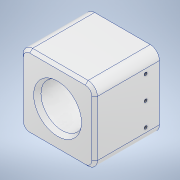
# Autodesk Inventor part: Temperierblock
Saved by Autodesk Inventor 2021 (Build 250183000, 183)
## iProperties
Created: 2021-04-25
Part Number: Temperierblock
Material: Aluminium 6061
Document SubType Name: Modeling
Designer: Sebastian Seewald
Density: 2.7 g/cm^3
Appearance: Aluminium - flach
Mass: 877.287 g
Surface Area: 506.723 cm^2
Volume: 324.921 cm^3
Author: Sebastian Seewald
Autodesk Inventor part; units mm, degrees
note: some values were not read from the file. Chosen so that the rebuilt part matches the saved one: pattern direction of "Rechteckige Anordnung1".
ref_plane "YZ Plane" through (0, 0, 0) normal (1, 0, 0) x (0, 1, 0)
ref_plane "XZ Plane" through (0, 0, 0) normal (0, 1, 0) x (-1, 0, 0)
ref_plane "XY Plane" through (0, 0, 0) normal (0, 0, 1) x (1, 0, 0)
sketch "Skizze1" plane through (0, 0, 0) normal (0, 0, 1) x (1, 0, 0)
  line L0 (-40, 40) -> (40, 40)
  line L1 (40, 40) -> (40, -40)
  line L2 (40, -40) -> (-40, -40)
  line L3 (-40, -40) -> (-40, 40)
  line L4 (-40, 40) -> (40, -40) construction
  line L5 (40, 40) -> (-40, -40) construction
  point P0 (0, 0)
  dimension "d0" = 80
  dimension "d1" = 80
  constraints: 12 end point, 2 midpoint, 2 parallel, 1 horizontal, 1 perpendicular
  measures "d0" distance of L0.start L0.end
  measures "d1" distance of L2.end L0.start
extrude "Extrusion1" add sketch "Skizze1" along normal blind 70
sketch "Skizze2" plane through (0, 0, 70) normal (0, 0, 1) x (1, 0, 0)
  circle A0 centre (0, 0) radius 22.95
  dimension "d4" = 45.9
  constraints: 1 centre point, 1 coincident
  measures "d4" diameter of A0
extrude "Extrusion2" cut sketch "Skizze2" against normal blind 60
chamfer "Fase1" distance 5 angle 30 1 edges at (-22.95, 0, 70) measured on face at (22.8756, -1.8467, 30)
fillet "Rundung2" radius 10 4 edges at (40, -40, 35) (40, 40, 35) (-40, -40, 35) (-40, 40, 35)
sketch "Skizze4" plane through (0, 0, 0) normal (0, 0, -1) x (-1, 0, 0)
  line L0 (40, 30) -> (40, -30) projected
  line L1 (-30, 40) -> (30, 40) projected
  point P0 (0, 0)
  point P1 (33, 33)
  dimension "d38" = 7
  dimension "d39" = 7
  measures "d38" distance from line of point (33, 33) L0
  measures "d39" distance from line of L1 point (33, 33)
hole "Bohrung1" at (-33, 33, 0) direction (0, 0, 1) diameter 3.242 depth 18 tip angle 118 thread size "M4x0.7" class "6H" standard "ISO Metric profile"
pattern_linear "Rechteckige Anordnung1" count 2 spacing 66 along (1, 0, 0) count 2 spacing 66 along (0, -1, 0) of "Bohrung1" first direction both ways yes
chamfer "Fase2" distance 3 angle 45 8 edges at (0, -40, 70) (37.0711, -37.0711, 70) (40, 0, 70) (37.0711, 37.0711, 70) (0, 40, 70) (-37.0711, 37.0711, 70) (-40, 0, 70) (-37.0711, -37.0711, 70)
sketch "Skizze8" plane through (0, 0, 0) normal (0, 0, -1) x (-1, 0, 0)
  point P0 (0, 0)
  point P1 (-25, -25)
  point P2 (-25, 25)
  point P3 (25, 25)
  point P4 (25, -25)
  dimension "d75" = 25
  dimension "d76" = 25
  dimension "d84" = 25
  dimension "d85" = 25
  dimension "d86" = 25
  dimension "d87" = 25
  dimension "d88" = 25
  dimension "d89" = 25
  measures "d75" horizontal distance of point (0, 0) point (-25, -25)
  measures "d76" horizontal distance of point (0, 0) point (-25, -25)
  measures "d84" horizontal distance of point (0, 0) point (-25, 25)
  measures "d85" horizontal distance of point (0, 0) point (-25, 25)
  measures "d86" horizontal distance of point (0, 0) point (25, 25)
  measures "d87" horizontal distance of point (0, 0) point (25, 25)
  measures "d88" horizontal distance of point (0, 0) point (25, -25)
  measures "d89" horizontal distance of point (0, 0) point (25, -25)
hole "Bohrung3" at (25, -25, 0) at (25, 25, 0) at (-25, 25, 0) at (-25, -25, 0) direction (0, 0, 1) diameter 8 depth 60 tip angle 118
sketch "Skizze10" plane through (0, 0, 0) normal (0, 0, -1) x (-1, 0, 0)
  point P0 (0, 0)
  point P1 (-30, 0)
  point P2 (30, 0)
  dimension "d97" = 30
  dimension "d98" = 30
  constraints: 2 horizontal alignment
  measures "d97" distance of point (0, 0) point (-30, 0)
  measures "d98" distance of point (0, 0) point (30, 0)
hole "Bohrung5" at (30, 0, 0) at (-30, 0, 0) direction (0, 0, 1) diameter 5.1 depth 50 tip angle 118
sketch "Skizze12" plane through (40, -30, 0) normal (1, 0, 0) x (0, 0, -1)
  point P0 (0, 30)
  point P1 (-15, 5)
  point P2 (-15, 55)
  dimension "d108" = 25
  dimension "d109" = 25
  dimension "d110" = 15
  dimension "d111" = 15
  measures "d108" vertical distance of point (0, 30) point (-15, 5)
  measures "d109" vertical distance of point (0, 30) point (-15, 55)
  measures "d110" horizontal distance of point (0, 30) point (-15, 5)
  measures "d111" horizontal distance of point (0, 30) point (-15, 55)
hole "Bohrung6" at (40, -25, 15) at (40, 25, 15) direction (-1, 0, 0) diameter 3.242 depth 13 tip angle 118 thread size "M4x0.7" class "6H" standard "ISO Metric profile"
sketch "Skizze13" plane through (-40, -30, 0) normal (-1, 0, 0) x (0, 0, 1)
  point P0 (0, 30)
  point P1 (15, 55)
  point P2 (15, 5)
  dimension "d119" = 25
  dimension "d120" = 25
  dimension "d121" = 15
  dimension "d122" = 15
  measures "d119" vertical distance of point (0, 30) point (15, 55)
  measures "d120" vertical distance of point (0, 30) point (15, 5)
  measures "d121" horizontal distance of point (0, 30) point (15, 5)
  measures "d122" horizontal distance of point (0, 30) point (15, 55)
hole "Bohrung7" at (-40, 25, 15) at (-40, -25, 15) direction (1, 0, 0) diameter 3.242 depth 13 tip angle 118 thread size "M4x0.7" class "6H" standard "ISO Metric profile"
sketch "Skizze14" plane through (-40, -30, 0) normal (-1, 0, 0) x (0, 0, 1)
  point P0 (0, 30)
  point P1 (15, 30)
  dimension "d130" = 15
  dimension "d131" = 0
  measures "d130" distance of point (0, 30) point (15, 30)
  measures "d131" vertical distance of point (0, 30) point (15, 30)
hole "Bohrung8" at (-40, 0, 15) direction (1, 0, 0) diameter 3.242 depth 10 tip angle 118 thread size "M4x0.7" class "6H" standard "ISO Metric profile"
sketch "Skizze15" plane through (40, -30, 0) normal (1, 0, 0) x (0, 0, -1)
  point P0 (0, 30)
  point P1 (-15, 30)
  dimension "d139" = 0
  dimension "d140" = 15
  measures "d139" vertical distance of point (0, 30) point (-15, 30)
  measures "d140" distance of point (0, 30) point (-15, 30)
hole "Bohrung9" at (40, 0, 15) direction (-1, 0, 0) diameter 3.242 depth 10 tip angle 118 thread size "M4x0.7" class "6H" standard "ISO Metric profile"
sketch "Skizze17" plane through (0, 0, 0) normal (0, 0, -1) x (-1, 0, 0)
  point P0 (0, 0)
  point P1 (0, -13.075)
  point P2 (0, 13.075)
  dimension "d148" = 13.075
  dimension "d149" = 13.075
  constraints: 2 vertical alignment
  measures "d148" distance of point (0, 0) point (0, -13.075)
  measures "d149" distance of point (0, 0) point (0, 13.075)
hole "Bohrung10" at (0, -13.075, 0) at (0, 13.075, 0) direction (0, 0, 1) diameter 2.459 depth 8 tip angle 118 thread size "M3x0.5" class "6H" standard "ISO Metric profile"
